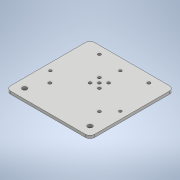
# Autodesk Inventor part: LRFマウント
Saved by Autodesk Inventor 2020 (Build 240168000, 168)
## iProperties
Part Number: LRFマウント
Material: 一般
Document SubType Name: Modeling
Designer: highs
Density: 1 g/cm^3
Appearance: 既定
Author: highs
Autodesk Inventor part; units mm, degrees
ref_plane "YZ Plane" through (0, 0, 0) normal (1, 0, 0) x (0, 1, 0)
ref_plane "XZ Plane" through (0, 0, 0) normal (0, 1, 0) x (-1, 0, 0)
ref_plane "XY Plane" through (0, 0, 0) normal (0, 0, 1) x (1, 0, 0)
sketch "スケッチ1" plane through (0, 0, 0) normal (0, 0, 1) x (1, 0, 0)
  line L0 (0, 0) -> (90, 0)
  line L1 (90, 0) -> (90, 90)
  line L2 (90, 90) -> (0, 90)
  line L3 (0, 90) -> (0, 0)
  line L4 (0, 10) -> (90, 10) construction
  circle A0 centre (10, 10) radius 2.5
  circle A1 centre (80, 10) radius 2.5
  circle A2 centre (18.5, 81.5) radius 1.6
  circle A3 centre (18.5, 28.5) radius 1.6
  circle A4 centre (71.5, 81.5) radius 1.6
  circle A5 centre (71.5, 28.5) radius 1.6
  line L5 (18.5, 81.5) -> (18.5, 28.5) construction
  line L6 (18.5, 28.5) -> (71.5, 28.5) construction
  line L7 (71.5, 28.5) -> (71.5, 81.5) construction
  line L8 (71.5, 81.5) -> (18.5, 81.5) construction
  line L9 (45, 90) -> (45, 0) construction
  line L10 (0, 55) -> (90, 55) construction
  line L11 (49.95, 50.05) -> (40.05, 50.05) construction
  line L12 (40.05, 50.05) -> (40.05, 59.95) construction
  line L13 (40.05, 59.95) -> (49.95, 59.95) construction
  line L14 (49.95, 59.95) -> (49.95, 50.05) construction
  line L15 (49.95, 50.05) -> (40.05, 59.95) construction
  line L16 (40.05, 50.05) -> (49.95, 59.95) construction
  circle A6 centre (49.95, 59.95) radius 1.6
  circle A7 centre (40.05, 59.95) radius 1.6
  circle A8 centre (49.95, 50.05) radius 1.6
  circle A9 centre (40.05, 50.05) radius 1.6
  circle A10 centre (45, 55) radius 1.6
  dimension "d0" = 5
  dimension "d1" = 10
  dimension "d2" = 10
  dimension "d3" = 10
  dimension "d4" = 90
  dimension "d5" = 90
  dimension "d12" = 3.2
  dimension "d21" = 53
  dimension "d23" = 53
  dimension "d33" = 55
  dimension "d34" = 3.2
  dimension "d35" = 9.9
  dimension "d36" = 9.9
  constraints: 34 end point, 11 centre point, 8 equal radius, 7 point on line, 6 perpendicular, 5 midpoint, 4 coincident, 4 parallel, 3 horizontal, 2 other
  measures "d0" diameter of A0
  measures "d1" distance from line of L3 A0.centre
  measures "d2" distance between parallel lines of L0 L4
  measures "d3" distance from line of L1 A1.centre
  measures "d4" distance of L0.start L0.end
  measures "d5" distance of L2.end L0.start
  measures "d12" diameter of A2
  measures "d21" distance between parallel lines of L6 L8
  measures "d23" distance of L7.end L5.start
  measures "d33" distance between parallel lines of L10 L0
  measures "d34" diameter of A6
  measures "d35" distance of L13.end L11.start
  measures "d36" distance of L12.end L13.end
extrude "押し出し1" add sketch "スケッチ1" along normal blind 3
sketch "スケッチ2" plane through (0, 0, 3) normal (0, 0, 1) x (1, 0, 0)
  line L0 (90, 90) -> (0, 90) construction
  line L1 (45, 90) -> (45, 0) construction
  line L2 (45, 77.4767) -> (82.4767, 40) construction
  line L3 (82.4767, 40) -> (45, 2.5233) construction
  line L4 (45, 2.5233) -> (7.5233, 40) construction
  line L5 (7.5233, 40) -> (45, 77.4767) construction
  line L6 (45, 77.4767) -> (45, 2.5233) construction
  line L7 (82.4767, 40) -> (7.5233, 40) construction
  line L8 (0, 0) -> (90, 0) construction
  circle A0 centre (82.4767, 40) radius 1.5
  circle A1 centre (45, 77.4767) radius 1.5
  circle A2 centre (45, 2.5233) radius 1.5 construction
  circle A3 centre (7.5233, 40) radius 1.5
  point P0 (45, 40)
  dimension "d27" = 53
  dimension "d28" = 90
  dimension "d29" = 40
  dimension "d30" = 3
  constraints: 14 end point, 4 centre point, 4 coincident, 3 equal radius, 3 midpoint, 2 parallel, 2 perpendicular, 1 point on line, 1 vertical
  measures "d27" distance of L2.start L2.end
  measures "d28" angle of L1 L7
  measures "d29" distance from line of L8 point (45, 40)
  measures "d30" diameter of A0
extrude "押し出し2" cut sketch "スケッチ2" against normal up to next
fillet "フィレット2" radius 5 4 edges at (90, 90, 1.5) (0, 90, 1.5) (90, 0, 1.5) (0, 0, 1.5)
sketch "スケッチ3" plane through (0, 0, 0) normal (0, 0, -1) x (-1, 0, 0)
  line L0 (-70, 65.05) -> (-20, 65.05)
  line L1 (-20, 65.05) -> (-20, 44.95)
  line L2 (-20, 44.95) -> (-70, 44.95)
  line L3 (-70, 44.95) -> (-70, 65.05)
  circle A0 centre (-45, 55) radius 1.6 projected
  line L4 (-70, 65.05) -> (-20, 44.95) construction
  line L5 (-20, 65.05) -> (-70, 44.95) construction
  point P0 (0, 0)
  dimension "d38" = 20.1
  dimension "d39" = 50
  constraints: 12 end point, 2 midpoint, 2 parallel, 1 horizontal, 1 perpendicular
  measures "d38" distance of L2.end L0.start
  measures "d39" distance of L0.start L0.end
extrude "押し出し3" cut sketch "スケッチ3" against normal blind 1
fillet "フィレット3" radius 2 4 edges at (70, 65.05, 0.5) (20, 65.05, 0.5) (20, 44.95, 0.5) (70, 44.95, 0.5)
